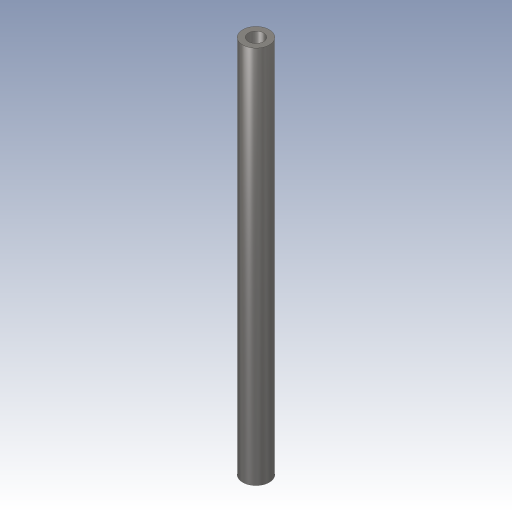
# Autodesk Inventor part: BT009_huenin20_23
Saved by Autodesk Inventor 2023.3 (Build 273359000, 359)
## iProperties
Company: HTBLA Kaindorf
RuleStatus: InUse
Created: 2023-09-19
Part Number: BT009_huenin20_23
Project: Fiberprinter-Hotend
Material: Edelstahl
Description: Fiber_führung
Document SubType Name: Modeling
Designer: huenin20
Density: 8 g/cm^3
Appearance: Halbpoliert
Mass: 0.0207345 g
Surface Area: 0.350759 cm^2
Volume: 0.00259181 cm^3
AfterDocNew0: iProperties-Editor_aufrufen
Author: nicob
Keywords: 2023
Autodesk Inventor part; units mm, degrees
ref_plane "YZ Plane" through (0, 0, 0) normal (1, 0, 0) x (0, 1, 0)
ref_plane "XZ Plane" through (0, 0, 0) normal (0, 1, 0) x (-1, 0, 0)
ref_plane "XY Plane" through (0, 0, 0) normal (0, 0, 1) x (1, 0, 0)
sketch "Skizze6" plane through (0, 0, 0) normal (0, 0, 1) x (1, 0, 0)
  circle A0 centre (0, 0) radius 0.2
  circle A1 centre (0, 0) radius 0.35
  dimension "d30" = 0.7
  dimension "d31" = 0.4
  constraints: 2 centre point, 2 coincident
  measures "d30" diameter of A1
  measures "d31" diameter of A0
extrude "Extrusion4" add sketch "Skizze6" along normal blind 10
